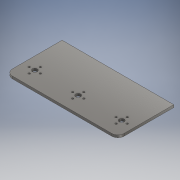
# Autodesk Inventor part: laterales2
Saved by Autodesk Inventor 2018 (Build 220112000, 112)
## iProperties
Created: 2019-04-03
Part Number: laterales2
Material: Acero, galvanizado
Document SubType Name: Modeling
Designer: Victor Hernandez
Density: 7.85 g/cm^3
Appearance: Galvanizado
Author: Victor Hernandez
Autodesk Inventor part; units mm, degrees
ref_plane "YZ Plane" through (0, 0, 0) normal (1, 0, 0) x (0, 1, 0)
ref_plane "XZ Plane" through (0, 0, 0) normal (0, 1, 0) x (-1, 0, 0)
ref_plane "XY Plane" through (0, 0, 0) normal (0, 0, 1) x (1, 0, 0)
sketch "Boceto1" plane through (0, 0, 0) normal (0, 0, 1) x (1, 0, 0)
  line L0 (-40, -22.5) -> (40, -22.5)
  line L1 (45, -17.5) -> (45, 22.5)
  line L2 (45, 22.5) -> (-45, 22.5)
  line L3 (-45, 22.5) -> (-45, -17.5)
  line L4 (-45, -22.5) -> (45, 22.5) construction
  line L5 (45, -22.5) -> (-45, 22.5) construction
  circle A0 centre (35, -9.5) radius 2
  circle A1 centre (35, -5) radius 0.75
  circle A2 centre (30.5, -9.5) radius 0.75
  circle A3 centre (35, -14) radius 0.75
  circle A4 centre (39.5, -9.5) radius 0.75
  circle A5 centre (0, -9.5) radius 2
  line L6 (0, -9.5) -> (4.5, -9.5) construction
  line L7 (0, -9.5) -> (4.5, -9.5) construction
  circle A6 centre (0, -5) radius 0.75
  circle A7 centre (4.5, -9.5) radius 0.75
  circle A8 centre (-4.5, -9.5) radius 0.75
  circle A9 centre (0, -14) radius 0.75
  line L8 (-45, -17.5) -> (-45, -9.5)
  circle A10 centre (-35, -9.5) radius 2
  line L9 (-35, -9.5) -> (-30.5, -9.5) construction
  line L10 (-35, -9.5) -> (-30.5, -9.5) construction
  line L11 (-35, -9.5) -> (-30.5, -9.5) construction
  circle A11 centre (-35, -5) radius 0.75
  circle A12 centre (-30.5, -9.5) radius 0.75
  circle A13 centre (-35, -14) radius 0.75
  circle A14 centre (-39.5, -9.5) radius 0.75
  arc A15 (-45, -17.5) -> (-40, -22.5) centre (-40, -17.5) ccw
  arc A16 (40, -22.5) -> (45, -17.5) centre (40, -17.5) ccw
  point P0 (0, 0)
  dimension "d0" = 90
  dimension "d1" = 45
  dimension "d4" = 4
  dimension "d6" = 1.5
  dimension "d9" = 1.5
  dimension "d10" = 1.5
  dimension "d14" = 4
  dimension "d20" = 1.5
  dimension "d21" = 1.5
  dimension "d22" = 1.5
  dimension "d24" = 1.5
  dimension "d25" = 13
  dimension "d27" = 4
  dimension "d30" = 4.5
  dimension "d34" = 1.5
  dimension "d35" = 1.5
  dimension "d36" = 1.5
  dimension "d38" = 1.5
  dimension "d40" = 5
  constraints: 24 end point, 17 centre point, 6 horizontal, 6 point on line, 4 point on circle, 4 tangent, 2 coincident, 2 midpoint, 2 parallel, 1 equal radius, 1 perpendicular
  measures "d0" distance of L2.end L1.end
  measures "d1" distance of L1.end L5.start
  measures "d4" diameter of A0
  measures "d6" diameter of A1
  measures "d9" diameter of A2
  measures "d10" diameter of A3
  measures "d14" diameter of A5
  measures "d20" diameter of A6
  measures "d21" diameter of A7
  measures "d22" diameter of A8
  measures "d24" diameter of A9
  measures "d25" distance of L4.start L8.end
  measures "d27" diameter of A10
  measures "d30" distance of L9.start L9.end
  measures "d34" diameter of A11
  measures "d35" diameter of A12
  measures "d36" diameter of A13
  measures "d38" diameter of A14
  measures "d40" radius of A15
extrude "Extrusión1" add sketch "Boceto1" along normal blind 2
